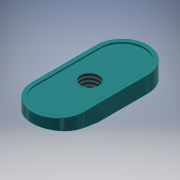
# Autodesk Inventor part: Lopez_LeftClamp
Saved by Autodesk Inventor 2018 (Build 220112000, 112)
## iProperties
Created: 2018-02-08
Part Number: Lopez_LeftClamp
Material: Polypropylene
Document SubType Name: Modeling
Designer: clopez06
Density: 0.899 g/cm^3
Appearance: Smooth - Ash
Author: clopez06
Autodesk Inventor part; units mm, degrees
ref_plane "YZ Plane" through (0, 0, 0) normal (1, 0, 0) x (0, 1, 0)
ref_plane "XZ Plane" through (0, 0, 0) normal (0, 1, 0) x (-1, 0, 0)
sketch "Sketch1" plane through (0, 0, 0) normal (0, 1, 0) x (-1, 0, 0)
  arc A0 (8.89, 11.1125) -> (-8.89, 11.1125) centre (0, 11.1125) ccw
  line L0 (-8.89, 0) -> (8.89, 0)
  arc A1 (-8.89, -11.1125) -> (8.89, -11.1125) centre (0, -11.1125) ccw
  line L1 (8.89, 11.1125) -> (8.89, -11.1125)
  line L2 (-8.89, 11.1125) -> (-8.89, -11.1125)
  point P0 (0, 0)
  constraints: 6 end point, 4 point on circle, 2 centre point, 2 tangent, 1 horizontal, 1 parallel, 1 symmetric about line, 1 vertical, 1 other
extrude "Extrusion1" add sketch "Sketch1" along normal blind 5.588
sketch "Sketch2" plane through (0, 5.588, 0) normal (0, 1, 0) x (1, 0, 0)
  arc A0 (-7.62, -11.1125) -> (7.62, -11.1125) centre (0, -11.1125) ccw
  arc A1 (7.62, 11.1125) -> (-7.62, 11.1125) centre (0, 11.1125) ccw
  line L0 (-7.62, -11.1125) -> (-7.62, 11.1125)
  line L1 (7.62, -11.1125) -> (7.62, 11.1125)
  line L2 (8.89, -11.1125) -> (8.89, 11.1125) projected
  line L3 (-8.89, 11.1125) -> (-8.89, -11.1125) projected
  arc A2 (-8.89, -11.1125) -> (8.89, -11.1125) centre (0, -11.1125) ccw projected
  point P0 (0, 0)
  dimension "d32" = 1.27
  dimension "d33" = 1.27
  dimension "d34" = 1.27
  dimension "d36" = 22.225
  dimension "d37" = 22.225
  dimension "d38" = 22.225
  constraints: 4 end point, 4 point on circle, 2 centre point, 2 tangent, 1 parallel, 1 vertical
  measures "d32" distance between parallel lines of L1 L2
  measures "d33" distance between parallel lines of L3 L0
  measures "d34" radial gap between concentric circles of A0 A2
  measures "d36" distance of A1.centre A0.centre
  measures "d37" distance of L0.start L0.end
  measures "d38" distance of L1.start L1.end
extrude "Extrusion2" cut sketch "Sketch2" against normal blind 0.508
sketch "Sketch3" plane through (0, 5.08, 0) normal (0, 1, 0) x (1, 0, 0)
  circle A0 centre (0, 0) radius 3.175
  point P0 (0, 0)
  dimension "d10" = 6.35
  constraints: 1 centre point, 1 coincident
  measures "d10" diameter of A0
hole "Hole1" at (0, 5.08, 0) direction (0, -1, 0) diameter 6.35 end through all
thread "Thread1" size "1/4-20 UNC" class "1B" standard "ANSI Unified Screw Threads" full length
sketch "Sketch4" plane through (8.89, 0, 11.1125) normal (1, 0, 0) x (0, 0, -1)
  line L0 (5.0165, 0) -> (-12.6241, 2.794)
  line L1 (-12.6241, 2.794) -> (-8.89, 2.2026)
  line L2 (-8.89, 0) -> (-8.89, 5.588) projected
  line L3 (-8.89, 2.2026) -> (-8.89, 0)
  line L4 (5.0165, 0) -> (-8.89, 0)
  line L5 (-8.89, 2.2026) -> (5.0165, 0)
  point P0 (11.1125, 0)
  dimension "d29" = 9
  dimension "d30" = 6.096
  constraints: 10 end point, 2 point on line, 1 collinear, 1 perpendicular
  measures "d29" angle of L4 L0
  measures "d30" distance of L0.start point (11.113, 0)
extrude "Extrusion3" cut sketch "Sketch4" against normal through all
ref_plane "Work Plane1" through (0, -2.54, 0) normal (0, -1, 0) x (1, 0, 0)
sketch "Sketch5" plane through (0, -2.54, 0) normal (0, -1, 0) x (1, 0, 0)
  circle A0 centre (0, 13.716) radius 6.35
  line L0 (-5.5625, 10.6531) -> (5.5625, 16.7789)
  point P0 (0, 0)
  dimension "d23" = 12.7
  dimension "d31" = 13.716
  constraints: 2 end point, 2 point on circle, 1 centre point, 1 coincident, 1 midpoint
  measures "d23" diameter of A0
  measures "d31" distance of point (0, 0) A0.centre
revolve "Revolution1" cut sketch "Sketch5" angle 360 about axis through (-5.5625, -2.54, 10.6531) along (0.8759844, 0, 0.4823395) picked at (2.4961, 12.478) contours A0 L0
sketch "Sketch6" plane through (0, 0, 0) normal (0, -1, 0) x (1, 0, 0)
  circle A0 centre (0, -11.1125) radius 2.286
  point P0 (0, 0)
  dimension "d25" = 4.572
  dimension "d26" = 11.1125
  constraints: 1 centre point, 1 coincident
  measures "d25" diameter of A0
  measures "d26" distance of A0.centre point (0, 0)
extrude "Extrusion4" add sketch "Sketch6" along normal blind 1.27
body "Solid1"
